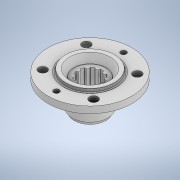
# Autodesk Inventor part: 65. Муфта вторичного вала
Saved by Autodesk Inventor 2021 (Build 250183000, 183)
## iProperties
Created: 2021-03-17
Part Number: 65. Муфта вторичного вала
Material: Типовые
Document SubType Name: Modeling
Designer: Данил
Density: 1 g/cm^3
Appearance: По умолчанию
Author: Данил
Autodesk Inventor part; units mm, degrees
ref_plane "YZ Plane" through (0, 0, 0) normal (1, 0, 0) x (0, 1, 0)
ref_plane "XZ Plane" through (0, 0, 0) normal (0, 1, 0) x (-1, 0, 0)
ref_plane "XY Plane" through (0, 0, 0) normal (0, 0, 1) x (1, 0, 0)
sketch "Эскиз1" plane through (0, 0, 0) normal (0, 0, 1) x (1, 0, 0)
  line L0 (0, 26.5) -> (0, -26.5)
  line L1 (17.5, -26.5) -> (22.9019, -26.5)
  line L2 (25.5, -22) -> (25.5, 5.5)
  line L3 (17.5, -26.5) -> (17.5, 16)
  line L4 (25.5, -22) -> (22.9019, -26.5)
  line L5 (26.5, 6.5) -> (31, 6.5)
  arc A0 (26.5, 6.5) -> (25.5, 5.5) centre (26.5, 5.5) ccw
  line L6 (31, 6.5) -> (31, 7.5)
  line L7 (31, 7.5) -> (29.5, 8.366)
  line L8 (29.5, 8.366) -> (29.5, 11)
  line L9 (31.5, 13) -> (60, 13)
  arc A1 (31.5, 13) -> (29.5, 11) centre (31.5, 11) ccw
  line L10 (60, 13) -> (60, 22.5)
  line L11 (60, 22.5) -> (38, 22.5)
  line L12 (38, 22.5) -> (36.5, 21.634)
  arc A2 (35, 22.5) -> (36.5, 21.634) centre (36, 22.5) ccw
  line L13 (35, 22.5) -> (35, 26)
  line L14 (34.7113, 26.5) -> (29.0622, 26.5)
  line L15 (29.0622, 26.5) -> (23.1443, 16.25)
  line L16 (22.7113, 16) -> (17.5, 16)
  arc A3 (22.7113, 16) -> (23.1443, 16.25) centre (22.7113, 16.5) ccw
  line L17 (35, 26) -> (34.7113, 26.5)
  point P0 (0, 0)
  point P1 (0, 0)
  point P2 (25.5, -26.5)
  point P3 (25.5, 6.5)
  point P4 (35, 26.5)
  point P5 (23, 16)
  dimension "d0" = 53
  dimension "d1" = 35
  dimension "d2" = 51
  dimension "d3" = 4.5
  dimension "d4" = 30
  dimension "d5" = 1
  dimension "d7" = 33
  dimension "d8" = 1
  dimension "d9" = 30
  dimension "d10" = 2
  dimension "d11" = 59
  dimension "d12" = 62
  dimension "d13" = 9.5
  dimension "d14" = 30
  dimension "d15" = 1
  dimension "d16" = 120
  dimension "d17" = 70
  dimension "d18" = 4
  dimension "d19" = 30
  dimension "d20" = 10.5
  dimension "d21" = 0.5
  dimension "d22" = 46
  dimension "d23" = 0.5
  dimension "d24" = 30
  constraints: 36 end point, 8 point on circle, 8 point on line, 8 tangent, 7 vertical, 5 horizontal, 4 centre point, 3 coincident, 3 horizontal alignment, 1 midpoint, 1 perpendicular
  measures "d0" distance of L0.start L0.end
  measures "d1" diameter of L3 L0
  measures "d2" diameter of point (25.5, 6.5) L0
  measures "d3" distance of L2.start point (25.5, -26.5)
  measures "d4" angle of L2 L4
  measures "d5" radius of A0
  measures "d7" distance between parallel lines of L1 L5
  measures "d8" distance of L5.end L6.end
  measures "d9" angle of L5 L7
  measures "d10" radius of A1
  measures "d11" diameter of L8 L0
  measures "d12" diameter of L6 L0
  measures "d13" distance of L9.end L10.end
  measures "d14" angle of L11 L12
  measures "d15" radius of A2
  measures "d16" diameter of L10 L0
  measures "d17" diameter of L13 L0
  measures "d18" distance from line of point (35, 26.5) L11
  measures "d19" angle of L13 L15
  measures "d20" distance from line of point (23, 16) L14
  measures "d21" radius of A3
  measures "d22" diameter of point (23, 16) L0
  measures "d23" distance of L13.end point (35, 26.5)
  measures "d24" angle of L13 L17
revolve "Вращение1" add sketch "Эскиз1" angle 360 about axis through (0, 26.5, 0) along (0, -1, 0)
sketch "Эскиз2" plane through (0, 22.5, 0) normal (0, 1, 0) x (1, 0, 0)
  circle A0 centre (0, 0) radius 48 construction
  circle A1 centre (-36.434, 31.25) radius 6
  line L0 (-36.434, 31.25) -> (-36.434, -31.25) construction
  circle A2 centre (-36.434, -31.25) radius 6
  circle A3 centre (36.434, 31.25) radius 6
  circle A4 centre (36.434, -31.25) radius 6
  circle A5 centre (0, -48) radius 4
  circle A6 centre (0, 48) radius 4
  dimension "d26" = 96
  dimension "d27" = 12
  dimension "d28" = 62.5
  dimension "d29" = 8
  constraints: 7 centre point, 6 point on circle, 4 equal radius, 2 coincident, 2 end point, 2 horizontal alignment, 2 vertical alignment, 1 vertical
  measures "d26" diameter of A0
  measures "d27" diameter of A1
  measures "d28" distance of L0.start L0.end
  measures "d29" diameter of A5
extrude "Выдавливание1" cut sketch "Эскиз2" against normal through all
thread "Резьба1" size "M12x1.25" class "6H" standard "ISO Metric profile" length 7.4
thread "Резьба2" size "M12x1.25" class "6H" standard "ISO Metric profile" length 7.4
thread "Резьба3" size "M12x1.25" class "6H" standard "ISO Metric profile" length 7.4
thread "Резьба4" size "M12x1.25" class "6H" standard "ISO Metric profile" length 7.4
thread "Резьба5" size "M8x1" class "6H" standard "ANSI Metric M Profile" length 7.4
thread "Резьба6" size "M8x1" class "6H" standard "ISO Metric profile" length 7.4
sketch "Эскиз3" plane through (0, 16, 0) normal (0, 1, 0) x (1, 0, 0)
  circle A0 centre (0, 0) radius 15
  circle A1 centre (0, 0) radius 17.5 projected
  circle A2 centre (0, 0) radius 17.5 construction
  line L0 (-2.5, -17.3205) -> (2.5, -17.3205) construction
  line L1 (8.1582, -15.482) -> (12.2033, -12.5431) construction
  line L2 (15.7002, -7.73) -> (17.2453, -2.9747) construction
  line L3 (17.2453, 2.9747) -> (15.7002, 7.73) construction
  line L4 (12.2033, 12.5431) -> (8.1582, 15.482) construction
  line L5 (2.5, 17.3205) -> (-2.5, 17.3205) construction
  line L6 (-8.1582, 15.482) -> (-12.2033, 12.5431) construction
  line L7 (-15.7002, 7.73) -> (-17.2453, 2.9747) construction
  line L8 (-17.2453, -2.9747) -> (-15.7002, -7.73) construction
  line L9 (-12.2033, -12.5431) -> (-8.1582, -15.482) construction
  line L10 (-2.5, -17.3205) -> (-2.9612, -14.7048)
  line L11 (-8.1582, -15.482) -> (-6.2476, -13.637)
  line L12 (2.5, -17.3205) -> (2.9612, -14.7048)
  line L13 (8.1582, -15.482) -> (6.2476, -13.637)
  line L14 (12.2033, -12.5431) -> (11.0389, -10.1559)
  line L15 (15.7002, -7.73) -> (13.07, -7.3603)
  line L16 (17.2453, -2.9747) -> (14.9002, -1.7277)
  line L17 (17.2453, 2.9747) -> (14.9002, 1.7277)
  line L18 (15.7002, 7.73) -> (13.07, 7.3603)
  line L19 (12.2033, 12.5431) -> (11.0389, 10.1559)
  line L20 (8.1582, 15.482) -> (6.2476, 13.637)
  line L21 (2.5, 17.3205) -> (2.9612, 14.7048)
  line L22 (-2.5, 17.3205) -> (-2.9612, 14.7048)
  line L23 (-8.1582, 15.482) -> (-6.2476, 13.637)
  line L24 (-12.2033, 12.5431) -> (-11.0389, 10.1559)
  line L25 (-15.7002, 7.73) -> (-13.07, 7.3603)
  line L26 (-17.2453, 2.9747) -> (-14.9002, 1.7277)
  line L27 (-17.2453, -2.9747) -> (-14.9002, -1.7277)
  line L28 (-15.7002, -7.73) -> (-13.07, -7.3603)
  line L29 (-12.2033, -12.5431) -> (-11.0389, -10.1559)
  point P0 (0, -17.3205)
  point P1 (10.1807, -14.0126)
  point P2 (16.4728, -5.3523)
  point P3 (16.4728, 5.3523)
  point P4 (10.1807, 14.0126)
  point P5 (0, 17.3205)
  point P6 (-10.1807, 14.0126)
  point P7 (-16.4728, 5.3523)
  point P8 (-16.4728, -5.3523)
  point P9 (-10.1807, -14.0126)
  point P10 (8.1582, -15.482)
  point P11 (6.2476, -13.637)
  point P12 (2.9612, -14.7048)
  point P13 (15.7002, -7.73)
  point P14 (13.07, -7.3603)
  point P15 (11.0389, -10.1559)
  point P16 (12.2033, -12.5431)
  point P17 (17.2453, 2.9747)
  point P18 (14.9002, 1.7277)
  point P19 (14.9002, -1.7277)
  point P20 (17.2453, -2.9747)
  point P21 (12.2033, 12.5431)
  point P22 (11.0389, 10.1559)
  point P23 (13.07, 7.3603)
  point P24 (15.7002, 7.73)
  point P25 (6.2476, 13.637)
  point P26 (8.1582, 15.482)
  point P27 (-6.2476, 13.637)
  point P28 (-2.9612, 14.7048)
  point P29 (-15.7002, 7.73)
  point P30 (-13.07, 7.3603)
  point P31 (-11.0389, 10.1559)
  point P32 (-12.2033, 12.5431)
  point P33 (-17.2453, -2.9747)
  point P34 (-14.9002, -1.7277)
  point P35 (-14.9002, 1.7277)
  point P36 (-17.2453, 2.9747)
  point P37 (-12.2033, -12.5431)
  point P38 (-11.0389, -10.1559)
  point P39 (-13.07, -7.3603)
  point P40 (-15.7002, -7.73)
  dimension "d44" = 30
  dimension "d45" = 5
  dimension "d48" = 360
  dimension "d50" = 100
  dimension "d51" = 56
  dimension "d54" = 360
  constraints: 60 end point, 4 point on circle, 1 centre point, 1 coincident, 1 horizontal, 1 midpoint, 1 vertical alignment, 102 other
  measures "d44" diameter of A0
  measures "d45" distance of L0.start L0.end
  measures "d50" angle of L0 L10
  measures "d51" angle of L10 L11
extrude "Выдавливание2" add sketch "Эскиз3" against normal up to surface (42.5 mm away) contours A0 L17 A1 L16 | A0 L19 A1 L18 | L15 A1 L14 A0 | A0 L21 A1 L20 | L13 A1 L12 A0 | A0 L23 A1 L22 | L10 A1 L11 A0 | A0 L25 A1 L24 | L29 A1 L28 A0 | A0 L27 A1 L26
fillet "Сопряжение1" radius 0.3 20 edges at (-2.5, -5.25, -17.3205) (-8.1582, -5.25, -15.482) (2.5, -5.25, -17.3205) (8.1582, -5.25, -15.482) (15.7002, -5.25, -7.73) (12.2033, -5.25, -12.5431) (17.2453, -5.25, -2.9747) (17.2453, -5.25, 2.9747) (15.7002, -5.25, 7.73) (12.2033, -5.25, 12.5431) (8.1582, -5.25, 15.482) (2.5, -5.25, 17.3205) (-2.5, -5.25, 17.3205) (-8.1582, -5.25, 15.482) (-12.2033, -5.25, 12.5431) (-15.7002, -5.25, 7.73) (-17.2453, -5.25, 2.9747) (-17.2453, -5.25, -2.9747) (-15.7002, -5.25, -7.73) (-12.2033, -5.25, -12.5431)
sketch "Эскиз4" plane through (0, -26.5, 0) normal (0, -1, 0) x (1, 0, 0)
  circle A0 centre (0, 0) radius 17.5 construction
  arc A1 (17.2065, 3.1917) -> (15.7964, 7.5316) centre (0, 0) ccw construction
  constraints: 1 centre point, 1 coincident, 1 concentric
sketch "Эскиз5" plane through (0, 0, 0) normal (0, 0, 1) x (1, 0, 0)
  line L0 (-17.5, -26.5) -> (17.5, -26.5) construction
  line L1 (15, -26.5) -> (15, 16) projected
  line L2 (17.5, -26.5) -> (15, -25.0566)
  line L3 (-22.9019, -26.5) -> (22.9019, -26.5) projected
  line L4 (0, -37.1) -> (0, 37.1) projected
  point P0 (0, 0)
  dimension "d59" = 30
  constraints: 2 end point, 1 point on line
  measures "d59" angle of L0 L2
revolve "Вращение2" cut sketch "Эскиз5" angle 360 about axis through (0, -10, 0) along (0, 1, 0)
